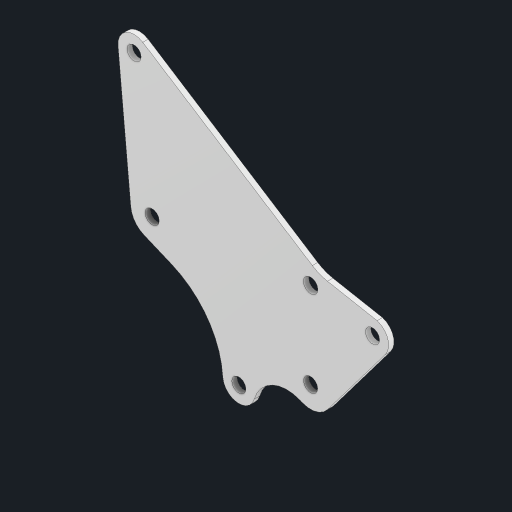
# Autodesk Inventor part: pod_gusset
Saved by Autodesk Inventor 2024 (Build 280153000, 153)
## iProperties
Created: 2023-08-18
Part Number: pod_gusset
Material: Acetal Resin, White
Document SubType Name: Modeling
Designer: Averey
Density: 1.425 g/cm^3
Appearance: Smooth - White
Author: Averey
Autodesk Inventor part; units mm, degrees
ref_plane "YZ Plane" through (0, 0, 0) normal (1, 0, 0) x (0, 1, 0)
ref_plane "XZ Plane" through (0, 0, 0) normal (0, 1, 0) x (-1, 0, 0)
ref_plane "XY Plane" through (0, 0, 0) normal (0, 0, 1) x (1, 0, 0)
sketch "Sketch3" plane through (0, 0, 0) normal (0, 0, 1) x (1, 0, 0)
  circle A0 centre (-54.2469, 21.2925) radius 2.0955
  arc A1 (-60.5679, 20.687) -> (-56.6908, 15.4316) centre (-54.2469, 21.2925) ccw
  arc A2 (-9.8006, -4.121) -> (-2.2878, -2.0849) centre (-7.3567, 1.7399) ccw
  arc A3 (-57.0411, 64.6274) -> (-64.3493, 60.162) centre (-59.6085, 60.6162) ccw
  circle A4 centre (-59.6085, 60.6162) radius 2.0955
  circle A5 centre (-7.3493, 27.1667) radius 2.15
  circle A6 centre (-7.3493, 27.1667) radius 2.0955
  arc A7 (-33.3475, -9.28) -> (-24.0182, -10.3106) centre (-28.5939, -8.9899) ccw
  circle A8 centre (-28.5939, -8.9899) radius 2.0955
  line L0 (-64.3493, 60.162) -> (-60.5679, 20.687)
  arc A9 (-10.5052, -3.8271) -> (-24.0182, -10.3106) centre (-14.3701, -13.0956) ccw
  arc A10 (-33.3475, -9.28) -> (-48.497, 12.0149) centre (-58.0042, -10.7848) ccw
  line L1 (-9.8006, -4.121) -> (-10.5052, -3.8271)
  line L2 (-48.497, 12.0149) -> (-56.6908, 15.4316)
  circle A11 centre (-7.3567, 1.7399) radius 2.0955
  line L3 (-2.3615, 30.7218) -> (12.3103, 27.9571)
  line L4 (-57.0411, 64.6274) -> (-6.8563, 32.5056)
  arc A12 (-6.8563, 32.5056) -> (-2.3615, 30.7218) centre (-0.0098, 43.2022) ccw
  circle A13 centre (10.9669, 23.388) radius 2.0955
  arc A14 (14.7685, 20.5194) -> (11.3785, 28.1327) centre (10.9669, 23.388) ccw
  line L5 (14.7685, 20.5194) -> (-2.2878, -2.0849)
  point P0 (-1.412, -0.4923)
  point P1 (-2.1133, -1.8418)
  point P2 (-2.622, -2.4915)
  dimension "d25" = 4.191
  dimension "d28" = 12.7
  dimension "d29" = 4.191
  dimension "d31" = 9.525
  dimension "d47" = 12.7
  dimension "d48" = 4.191
  dimension "d49" = 9.525
  constraints: 20 point on circle, 17 tangent, 15 centre point, 12 end point, 6 coincident, 1 point on line, 6 other
  measures "d25" diameter of A0
  measures "d28" diameter of A2
  measures "d29" diameter of A4
  measures "d31" diameter of A7
  measures "d47" radius of A12
  measures "d48" diameter of A13
  measures "d49" diameter of A14
extrude "Extrusion2" add sketch "Sketch3" along normal blind 1.5875 contours L0 A3 L4 A12 L3 A14 L5 A2 L1 A9 A7 A10 L2 A1
body "Solid2"
